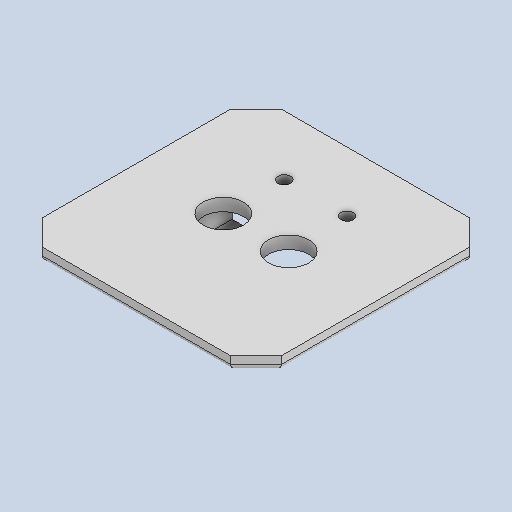
# Autodesk Inventor part: TutupAtas
Saved by Autodesk Inventor 2026.2 (Build 302298010, 298A)
## iProperties
Created: 2026-05-27
Part Number: TutupAtas
Material: Generic
Document SubType Name: Modeling
Designer: rizky
Density: 1 g/cm^3
Appearance: Default
Author: rizky
Autodesk Inventor part; units mm, degrees
ref_plane "YZ Plane" through (0, 0, 0) normal (1, 0, 0) x (0, 1, 0)
ref_plane "XZ Plane" through (0, 0, 0) normal (0, 1, 0) x (-1, 0, 0)
ref_plane "XY Plane" through (0, 0, 0) normal (0, 0, 1) x (1, 0, 0)
sketch "Sketch1" plane through (0, 0, 0) normal (0, 1, 0) x (-1, 0, 0)
  line L0 (0, 0) -> (95, 0)
  line L1 (95, 0) -> (95, -95)
  line L2 (95, -95) -> (0, -95)
  line L3 (0, -95) -> (0, 0)
  dimension "d0" = 95
  dimension "d1" = 95
  constraints: 8 end point, 2 parallel, 1 horizontal, 1 perpendicular
  measures "d0" distance of L1.end L2.end
  measures "d1" distance of L0.end L1.end
extrude "Extrusion1" add sketch "Sketch1" along normal blind 5
chamfer "Chamfer1" distance 10 angle 45 4 edges at (0, 2.5, -95) (0, 2.5, 0) (-95, 2.5, 0) (-95, 2.5, -95)
sketch "Sketch2" plane through (0, 0, 0) normal (0, -1, 0) x (1, 0, 0)
  line L0 (-85, -95) -> (-95, -85) projected
  line L1 (-10, -95) -> (-85, -95) projected
  line L2 (0, -85) -> (-10, -95) projected
  line L3 (0, -10) -> (0, -85) projected
  line L4 (-10, 0) -> (0, -10) projected
  line L5 (-85, 0) -> (-10, 0) projected
  line L6 (-95, -10) -> (-85, 0) projected
  line L7 (-95, -85) -> (-95, -10) projected
  line L8 (-47.5, -95) -> (-47.5, -71.232)
  line L9 (-47.5, -71.232) -> (-35, -71.232)
  circle A0 centre (-35, -71.232) radius 2.5
  circle A1 centre (-60, -71.232) radius 2.5
  point P0 (0, 0)
  dimension "d7" = 23.768
  dimension "d9" = 12.5
  dimension "d15" = 5
  constraints: 4 end point, 2 centre point, 2 coincident, 1 horizontal, 1 midpoint, 1 symmetric about line, 1 vertical, 1 other
  measures "d7" distance of L8.start L8.end
  measures "d9" distance of L9.start L9.end
  measures "d15" diameter of A0
extrude "Extrusion2" cut sketch "Sketch2" against normal blind 5 contours A0 | A1
sketch "Sketch3" plane through (0, 0, 0) normal (0, -1, 0) x (1, 0, 0)
  circle A0 centre (-35, -71.232) radius 2.5 projected
  line L0 (-85, -95) -> (-95, -85) projected
  line L1 (-10, -95) -> (-85, -95) projected
  line L2 (0, -85) -> (-10, -95) projected
  line L3 (0, -10) -> (0, -85) projected
  line L4 (-10, 0) -> (0, -10) projected
  line L5 (-85, 0) -> (-10, 0) projected
  line L6 (-95, -10) -> (-85, 0) projected
  line L7 (-95, -85) -> (-95, -10) projected
  line L8 (-47.5, -95) -> (-47.5, -47.5)
  line L9 (-85, 0) -> (-10, 0) projected
  line L10 (-34.5, -47.5) -> (-60.5, -47.5)
  circle A1 centre (-34.5, -47.5) radius 8
  circle A2 centre (-60.5, -47.5) radius 8
  point P0 (0, 0)
  dimension "d17" = 47.5
  dimension "d18" = 26
  dimension "d19" = 16
  constraints: 4 end point, 2 centre point, 2 midpoint, 1 coincident, 1 horizontal, 1 perpendicular, 1 symmetric about line, 1 other
  measures "d17" distance of L8.end L8.start
  measures "d18" distance of L10.start L10.end
  measures "d19" diameter of A1
extrude "Extrusion3" cut sketch "Sketch3" against normal blind 5 contours A1 | A2
sketch "Sketch4" plane through (0, 0, 0) normal (0, -1, 0) x (1, 0, 0)
  circle A0 centre (-60.5, -47.5) radius 8 projected
  circle A1 centre (-34.5, -47.5) radius 8 projected
  circle A2 centre (-35, -71.232) radius 2.5 projected
  line L0 (-85, -95) -> (-95, -85) projected
  line L1 (-10, -95) -> (-85, -95) projected
  line L2 (0, -85) -> (-10, -95) projected
  line L3 (0, -10) -> (0, -85) projected
  line L4 (-10, 0) -> (0, -10) projected
  line L5 (-85, 0) -> (-10, 0) projected
  line L6 (-95, -10) -> (-85, 0) projected
  line L7 (-95, -85) -> (-95, -10) projected
  line L8 (-47.5, -95) -> (-47.5, -47.5)
  line L9 (-85, 0) -> (-10, 0) projected
  line L10 (-70, -57.5) -> (-25, -57.5)
  line L11 (-25, -57.5) -> (-25, -37.5)
  line L12 (-25, -37.5) -> (-70, -37.5)
  line L13 (-70, -37.5) -> (-70, -57.5)
  line L14 (-70, -57.5) -> (-25, -37.5) construction
  line L15 (-25, -57.5) -> (-70, -37.5) construction
  line L16 (-22, -34.5) -> (-22, -60.5)
  line L17 (-22, -60.5) -> (-73, -60.5)
  line L18 (-73, -60.5) -> (-73, -34.5)
  line L19 (-73, -34.5) -> (-22, -34.5)
  line L20 (-25, -57.5) -> (-25, -60.5)
  line L21 (-70, -57.5) -> (-70, -60.5)
  point P0 (0, 0)
  point P1 (-70, -60.5)
  dimension "d22" = 47.5
  dimension "d23" = 45
  dimension "d24" = 20
  dimension "d25" = 3
  constraints: 26 end point, 4 parallel, 4 perpendicular, 3 midpoint, 1 horizontal, 1 point on line, 1 symmetric about line, 3 other
  measures "d22" distance of L8.start L8.end
  measures "d23" distance of L12.end L11.end
  measures "d24" distance of L11.end L10.end
  measures "d25" distance between parallel lines of L11 L16
extrude "Extrusion4" add sketch "Sketch4" along normal blind 11.2 contours L20 L11 L12 L13 L21 L17 L18 L19 L16
sketch "Sketch5" plane through (0, -11.2, 0) normal (0, -1, 0) x (1, 0, 0)
  line L0 (-70, -37.5) -> (-25, -37.5) projected
  line L1 (-25, -37.5) -> (-25, -60.5) projected
  line L2 (-25, -60.5) -> (-22, -60.5) projected
  line L3 (-22, -60.5) -> (-22, -34.5) projected
  line L4 (-22, -34.5) -> (-73, -34.5) projected
  line L5 (-73, -34.5) -> (-73, -60.5) projected
  line L6 (-73, -60.5) -> (-70, -60.5) projected
  line L7 (-70, -60.5) -> (-70, -37.5) projected
  line L8 (-25, -60.5) -> (-70, -60.5)
  point P0 (0, 0)
  constraints: 2 end point, 1 horizontal
extrude "Extrusion5" add sketch "Sketch5" against normal blind 3 contours L0 L1 L8 L7
sketch "Sketch6" plane through (0, -11.2, 0) normal (0, -1, 0) x (1, 0, 0)
  line L0 (-25, -37.5) -> (-70, -37.5) projected
  line L1 (-70, -37.5) -> (-70, -60.5) projected
  line L2 (-25, -60.5) -> (-25, -37.5) projected
  line L3 (-70, -37.5) -> (-70, -39.25)
  line L4 (-70, -39.25) -> (-68, -39.25)
  circle A0 centre (-68, -39.25) radius 1.5
  line L5 (-47.5, -37.5) -> (-47.5, -39.5)
  circle A1 centre (-27, -39.25) radius 1.5
  line L6 (-73, -60.5) -> (-22, -60.5) projected
  line L7 (-47.5, -60.5) -> (-57.5, -60.5)
  line L8 (-57.5, -60.5) -> (-57.5, -52.5)
  line L9 (-57.5, -52.5) -> (-47.5, -52.5)
  line L10 (-47.5, -52.5) -> (-47.5, -60.5)
  line L11 (-37.5, -60.5) -> (-37.5, -52.5)
  line L12 (-37.5, -52.5) -> (-47.5, -52.5)
  point P0 (0, 0)
  dimension "d30" = 1.75
  dimension "d31" = 2
  dimension "d32" = 3
  dimension "d33" = 2
  dimension "d36" = 10
  dimension "d37" = 8
  constraints: 18 end point, 3 symmetric about line, 2 centre point, 2 midpoint, 2 parallel, 2 perpendicular, 1 coincident, 1 horizontal, 1 point on line, 1 vertical, 1 other
  measures "d30" distance of L0.end L3.end
  measures "d31" distance of L3.end L4.end
  measures "d32" diameter of A0
  measures "d33" distance of L5.start L5.end
  measures "d36" distance of L8.end L9.end
  measures "d37" distance of L7.end L8.end
extrude "Extrusion6" cut sketch "Sketch6" against normal blind 3 contours L6 L10 L12 L11 | L6 L8 L9 L10 | A0 | A1
fillet "Fillet1" radius 2 16 edges at (-90, 0, -5) (-95, 0, -47.5) (-47.5, 0, 0) (-5, 0, -5) (0, 0, -47.5) (-90, 0, -90) (-47.5, 0, -95) (-5, 0, -90) (-22, -11.2, -47.5) (-47.5, -11.2, -34.5) (-73, -11.2, -47.5) (-65.25, -11.2, -60.5) (-29.75, -11.2, -60.5) (-47.5, -11.2, -52.5) (-57.5, -11.2, -56.5) (-37.5, -11.2, -56.5)
body "Solid1"
